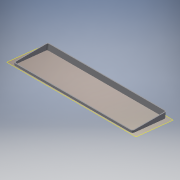
# Autodesk Inventor part: FullEnclosurePrototype2
Saved by Autodesk Inventor 2016 (Build 200138000, 138)
## iProperties
Created: 2021-04-06
Part Number: FullEnclosurePrototype2
Material: Generic
Document SubType Name: Modeling
Designer: Tom
Density: 1 g/cm^3
Appearance: Default
Author: Tom
Autodesk Inventor part; units mm, degrees
(part 1 of 3)
ref_plane "YZ Plane" through (0, 0, 0) normal (1, 0, 0) x (0, 1, 0)
ref_plane "XZ Plane" through (0, 0, 0) normal (0, 1, 0) x (-1, 0, 0)
ref_plane "XY Plane" through (0, 0, 0) normal (0, 0, 1) x (1, 0, 0)
ref_plane "Work Plane1" through (-46.4829, -22.3295, 9.2415) normal (0, 0.1062088, 0.9943439) x (-1, 0, 0)
sketch "Sketch1" plane through (-46.4829, -22.3295, 9.2415) normal (0, 0.1062088, 0.9943439) x (-1, 0, 0)
  line L0 (-256.8052, 108.1981) -> (-256.8112, -5.1571) projected
  ellipse E0 centre (-252.0612, -5.1574) end of major axis (-256.8112, -5.1571) minor radius 4.7231 (-256.8112, -5.1571) -> (-252.0615, -9.8805) ccw projected
  line L1 (-252.0615, -9.8805) -> (180.1885, -9.9036) projected
  ellipse E1 centre (180.1888, -5.1804) end of major axis (175.4388, -5.1802) minor radius 4.7231 (180.1885, -9.9036) -> (184.9388, -5.1807) ccw projected
  line L2 (184.9388, -5.1807) -> (184.9448, 108.1745) projected
  ellipse E2 centre (180.1948, 108.1748) end of major axis (175.4448, 108.175) minor radius 4.7231 (184.9448, 108.1745) -> (180.1951, 112.8979) ccw projected
  line L3 (180.1951, 112.8979) -> (-252.0549, 112.921) projected
  ellipse E3 centre (-252.0552, 108.1978) end of major axis (-256.8052, 108.1981) minor radius 4.7231 (-252.0549, 112.921) -> (-256.8052, 108.1981) ccw projected
  ellipse E4 centre (79.4979, 35.9093) end of major axis (79.2479, 35.9094) minor radius 0.2486 projected
  ellipse E5 centre (81.4737, -6.2143) end of major axis (81.0737, -6.2142) minor radius 0.3977 projected
  ellipse E6 centre (78.9337, -6.2141) end of major axis (78.5337, -6.2141) minor radius 0.3977 projected
  ellipse E7 centre (78.9345, 8.9397) end of major axis (78.5345, 8.9397) minor radius 0.3977 projected
  ellipse E8 centre (78.0659, 35.3197) end of major axis (77.8159, 35.3197) minor radius 0.2486 projected
  ellipse E9 centre (76.6341, 35.9095) end of major axis (76.3841, 35.9095) minor radius 0.2486 projected
  ellipse E10 centre (71.1058, 32.9386) end of major axis (70.3558, 32.9386) minor radius 0.7458 projected
  ellipse E11 centre (68.5655, 27.8874) end of major axis (66.5655, 27.8876) minor radius 1.9887 projected
  ellipse E12 centre (73.6455, 27.8872) end of major axis (72.7955, 27.8872) minor radius 0.8452 projected
  ellipse E13 centre (76.3937, -6.214) end of major axis (75.9937, -6.214) minor radius 0.3977 projected
  ellipse E14 centre (73.8537, -6.2139) end of major axis (73.4537, -6.2138) minor radius 0.3977 projected
  ellipse E15 centre (76.3945, 8.9398) end of major axis (75.9945, 8.9398) minor radius 0.3977 projected
  ellipse E16 centre (71.3137, -6.2137) end of major axis (70.9137, -6.2137) minor radius 0.3977 projected
  ellipse E17 centre (68.7745, 8.9402) end of major axis (68.3745, 8.9402) minor radius 0.3977 projected
  ellipse E18 centre (68.7737, -6.2136) end of major axis (68.3737, -6.2136) minor radius 0.3977 projected
  ellipse E19 centre (43.3737, -6.2122) end of major axis (42.9737, -6.2122) minor radius 0.3977 projected
  ellipse E20 centre (44.9851, 1.469) end of major axis (44.6101, 1.469) minor radius 0.3729 projected
  ellipse E21 centre (44.9852, 2.7318) end of major axis (44.6102, 2.7318) minor radius 0.3729 projected
  ellipse E22 centre (43.3745, 8.9416) end of major axis (42.9745, 8.9416) minor radius 0.3977 projected
  ellipse E23 centre (44.4855, 27.8887) end of major axis (43.6355, 27.8888) minor radius 0.8452 projected
  ellipse E24 centre (50.9937, -6.2126) end of major axis (50.5937, -6.2126) minor radius 0.3977 projected
  ellipse E25 centre (48.4537, -6.2125) end of major axis (48.0537, -6.2125) minor radius 0.3977 projected
  ellipse E26 centre (45.9137, -6.2124) end of major axis (45.5137, -6.2123) minor radius 0.3977 projected
  ellipse E27 centre (56.0737, -6.2129) end of major axis (55.6737, -6.2129) minor radius 0.3977 projected
  ellipse E28 centre (54.891, -1.1616) end of major axis (54.391, -1.1616) minor radius 0.4972 projected
  ellipse E29 centre (53.5337, -6.2128) end of major axis (53.1337, -6.2128) minor radius 0.3977 projected
  ellipse E30 centre (52.3511, 1.3642) end of major axis (51.8511, 1.3642) minor radius 0.4972 projected
  ellipse E31 centre (54.8911, 1.3641) end of major axis (54.3911, 1.3641) minor radius 0.4972 projected
  ellipse E32 centre (58.6137, -6.213) end of major axis (58.2137, -6.213) minor radius 0.3977 projected
  ellipse E33 centre (58.6145, 8.9408) end of major axis (58.2145, 8.9408) minor radius 0.3977 projected
  ellipse E34 centre (53.5345, 8.941) end of major axis (53.1345, 8.941) minor radius 0.3977 projected
  ellipse E35 centre (45.9145, 8.9414) end of major axis (45.5145, 8.9415) minor radius 0.3977 projected
  ellipse E36 centre (48.4545, 8.9413) end of major axis (48.0545, 8.9413) minor radius 0.3977 projected
  ellipse E37 centre (50.9945, 8.9412) end of major axis (50.5945, 8.9412) minor radius 0.3977 projected
  ellipse E38 centre (54.8913, 3.8897) end of major axis (54.3913, 3.8897) minor radius 0.4972 projected
  ellipse E39 centre (54.6455, 27.8882) end of major axis (53.7955, 27.8882) minor radius 0.8452 projected
  ellipse E40 centre (49.5655, 27.8885) end of major axis (47.5655, 27.8886) minor radius 1.9887 projected
  ellipse E41 centre (66.2337, -6.2135) end of major axis (65.8337, -6.2134) minor radius 0.3977 projected
  ellipse E42 centre (63.6937, -6.2133) end of major axis (63.2937, -6.2133) minor radius 0.3977 projected
  ellipse E43 centre (63.6945, 8.9405) end of major axis (63.2945, 8.9405) minor radius 0.3977 projected
  ellipse E44 centre (63.4855, 27.8877) end of major axis (62.6355, 27.8878) minor radius 0.8452 projected
  ellipse E45 centre (61.1537, -6.2132) end of major axis (60.7537, -6.2132) minor radius 0.3977 projected
  ellipse E46 centre (52.1058, 32.9396) end of major axis (51.3558, 32.9396) minor radius 0.7458 projected
  ellipse E47 centre (39.1207, -3.7491) end of major axis (38.8707, -3.7491) minor radius 0.2486 projected
  ellipse E48 centre (39.1206, -6.5967) end of major axis (38.8706, -6.5967) minor radius 0.2486 projected
  ellipse E49 centre (39.7138, -5.1729) end of major axis (39.4638, -5.1729) minor radius 0.2486 projected
  ellipse E50 centre (68.5666, 46.78) end of major axis (66.5666, 46.7801) minor radius 1.9887 projected
  ellipse E51 centre (73.6466, 46.7797) end of major axis (72.7966, 46.7798) minor radius 0.8452 projected
  ellipse E52 centre (80.091, 37.3331) end of major axis (79.841, 37.3331) minor radius 0.2486 projected
  ellipse E53 centre (79.498, 38.7569) end of major axis (79.248, 38.7569) minor radius 0.2486 projected
  ellipse E54 centre (76.6342, 38.7571) end of major axis (76.3842, 38.7571) minor radius 0.2486 projected
  ellipse E55 centre (78.066, 37.3332) end of major axis (76.716, 37.3333) minor radius 1.3424 projected
  ellipse E56 centre (78.0662, 39.3468) end of major axis (77.8162, 39.3468) minor radius 0.2486 projected
  ellipse E57 centre (49.5666, 46.781) end of major axis (47.5666, 46.7811) minor radius 1.9887 projected
  ellipse E58 centre (54.6466, 46.7807) end of major axis (53.7966, 46.7808) minor radius 0.8452 projected
  ellipse E59 centre (63.4866, 46.7803) end of major axis (62.6366, 46.7803) minor radius 0.8452 projected
  ellipse E60 centre (45.7567, 49.3068) end of major axis (45.0067, 49.3069) minor radius 0.7458 projected
  ellipse E61 centre (37.6889, -3.1593) end of major axis (37.4389, -3.1593) minor radius 0.2486 projected
  ellipse E62 centre (36.2568, -6.5966) end of major axis (36.0068, -6.5965) minor radius 0.2486 projected
  ellipse E63 centre (35.6638, -5.1727) end of major axis (35.4138, -5.1727) minor radius 0.2486 projected
  ellipse E64 centre (71.1068, 51.8311) end of major axis (70.3568, 51.8312) minor radius 0.7458 projected
  ellipse E65 centre (52.1068, 51.8321) end of major axis (51.3568, 51.8322) minor radius 0.7458 projected
  ellipse E66 centre (14.8827, 68.201) end of major axis (14.1327, 68.2011) minor radius 0.7458 projected
  ellipse E67 centre (13.6126, 65.6754) end of major axis (12.7626, 65.6755) minor radius 0.8452 projected
  ellipse E68 centre (20.7355, 27.89) end of major axis (19.8855, 27.89) minor radius 0.8452 projected
  ellipse E69 centre (22.0057, 30.4156) end of major axis (21.2557, 30.4156) minor radius 0.7458 projected
  ellipse E70 centre (21.0666, 46.7825) end of major axis (19.0666, 46.7826) minor radius 1.9887 projected
  ellipse E71 centre (29.1358, 68.974) end of major axis (28.8858, 68.974) minor radius 0.2486 projected
  ellipse E72 centre (23.7726, 65.6749) end of major axis (22.9226, 65.675) minor radius 0.8452 projected
  ellipse E73 centre (28.3543, 4.6021) end of major axis (27.6043, 4.6021) minor radius 0.7458 projected
  ellipse E74 centre (25.814, -0.4491) end of major axis (23.814, -0.449) minor radius 1.9887 projected
  ellipse E75 centre (20.734, -0.4488) end of major axis (19.884, -0.4488) minor radius 0.8452 projected
  ellipse E76 centre (30.5677, 68.3841) end of major axis (30.3177, 68.3841) minor radius 0.2486 projected
  ellipse E77 centre (5.2939, -3.3316) end of major axis (4.8939, -3.3316) minor radius 0.3977 projected
  ellipse E78 centre (7.8939, -3.3317) end of major axis (7.4939, -3.3317) minor radius 0.3977 projected
  ellipse E79 centre (5.5937, -6.9609) end of major axis (5.0937, -6.9609) minor radius 0.4972 (5.5937, -6.4638) -> (5.5937, -7.4581) ccw projected
  line L4 (7.5937, -6.4639) -> (5.5937, -6.4638) projected
  ellipse E80 centre (7.5937, -6.961) end of major axis (7.0937, -6.961) minor radius 0.4972 (7.5937, -7.4582) -> (7.5937, -6.4639) ccw projected
  line L5 (5.5937, -7.4581) -> (7.5937, -7.4582) projected
  ellipse E81 centre (9.994, -0.5477) end of major axis (9.594, -0.5476) minor radius 0.3977 projected
  ellipse E82 centre (9.1913, 41.712) end of major axis (8.9413, 41.712) minor radius 0.2486 projected
  ellipse E83 centre (9.1912, 39.6985) end of major axis (7.8412, 39.6985) minor radius 1.3424 projected
  ellipse E84 centre (7.7594, 41.1223) end of major axis (7.5094, 41.1223) minor radius 0.2486 projected
  ellipse E85 centre (10.623, 38.2746) end of major axis (10.373, 38.2746) minor radius 0.2486 projected
  ellipse E86 centre (9.1911, 37.6849) end of major axis (8.9411, 37.6849) minor radius 0.2486 projected
  ellipse E87 centre (9.3558, 32.9419) end of major axis (8.6058, 32.9419) minor radius 0.7458 projected
  line L6 (13.9437, -6.9117) -> (13.9438, -5.4202) projected
  ellipse E88 centre (13.4437, -6.9116) end of major axis (12.9437, -6.9116) minor radius 0.4972 (12.9437, -6.9116) -> (13.9437, -6.9117) ccw projected
  line L7 (12.9438, -5.4201) -> (12.9437, -6.9116) projected
  ellipse E89 centre (13.4438, -5.4201) end of major axis (12.9438, -5.4201) minor radius 0.4972 (13.9438, -5.4202) -> (12.9438, -5.4201) ccw projected
  ellipse E90 centre (11.2162, 39.6983) end of major axis (10.9662, 39.6984) minor radius 0.2486 projected
  ellipse E91 centre (37.6887, -7.1864) end of major axis (37.4387, -7.1864) minor radius 0.2486 projected
  ellipse E92 centre (37.6888, -5.1728) end of major axis (36.3388, -5.1728) minor radius 1.3424 projected
  ellipse E93 centre (30.894, -0.4493) end of major axis (30.044, -0.4493) minor radius 0.8452 projected
  ellipse E94 centre (25.8155, 27.8897) end of major axis (23.8155, 27.8898) minor radius 1.9887 projected
  ellipse E95 centre (30.8955, 27.8895) end of major axis (30.0455, 27.8895) minor radius 0.8452 projected
  ellipse E96 centre (22.0042, 2.0768) end of major axis (21.2542, 2.0768) minor radius 0.7458 projected
  ellipse E97 centre (-36.2645, 27.893) end of major axis (-37.1145, 27.8931) minor radius 0.8452 projected
  ellipse E98 centre (-34.9943, 30.4186) end of major axis (-35.7443, 30.4186) minor radius 0.7458 projected
  ellipse E99 centre (-28.6442, 32.9439) end of major axis (-29.3942, 32.9439) minor radius 0.7458 projected
  ellipse E100 centre (-31.1845, 27.8928) end of major axis (-33.1845, 27.8929) minor radius 1.9887 projected
  ellipse E101 centre (-26.7634, 46.7851) end of major axis (-27.6134, 46.7851) minor radius 0.8452 projected
  ellipse E102 centre (-15.9943, 30.4176) end of major axis (-16.7443, 30.4176) minor radius 0.7458 projected
  ellipse E103 centre (-17.2645, 27.892) end of major axis (-18.1145, 27.8921) minor radius 0.8452 projected
  ellipse E104 centre (-21.6834, 46.7848) end of major axis (-23.6834, 46.7849) minor radius 1.9887 projected
  ellipse E105 centre (-25.4933, 49.3106) end of major axis (-26.2433, 49.3107) minor radius 0.7458 projected
  ellipse E106 centre (-12.1845, 27.8918) end of major axis (-14.1845, 27.8919) minor radius 1.9887 projected
  ellipse E107 centre (-9.6442, 32.9429) end of major axis (-10.3942, 32.9429) minor radius 0.7458 projected
  ellipse E108 centre (-12.186, -0.447) end of major axis (-14.186, -0.4469) minor radius 1.9887 projected
  ellipse E109 centre (-28.6457, 4.6051) end of major axis (-29.3957, 4.6051) minor radius 0.7458 projected
  ellipse E110 centre (-31.186, -0.446) end of major axis (-33.186, -0.4459) minor radius 1.9887 projected
  ellipse E111 centre (-19.1432, 51.8359) end of major axis (-19.8932, 51.836) minor radius 0.7458 projected
  ellipse E112 centre (-7.106, -0.4473) end of major axis (-7.956, -0.4473) minor radius 0.8452 projected
  ellipse E113 centre (-6.4933, 49.3096) end of major axis (-7.2433, 49.3097) minor radius 0.7458 projected
  ellipse E114 centre (-7.7634, 46.7841) end of major axis (-8.6134, 46.7841) minor radius 0.8452 projected
  ellipse E115 centre (-0.2562, -5.4194) end of major axis (-0.7562, -5.4194) minor radius 0.4972 (0.2438, -5.4194) -> (-0.7562, -5.4194) ccw projected
  line L8 (0.2437, -6.9109) -> (0.2438, -5.4194) projected
  ellipse E116 centre (-0.2563, -6.9109) end of major axis (-0.7563, -6.9109) minor radius 0.4972 (-0.7563, -6.9109) -> (0.2437, -6.9109) ccw projected
  line L9 (-0.7562, -5.4194) -> (-0.7563, -6.9109) projected
  ellipse E117 centre (-2.6834, 46.7838) end of major axis (-4.6834, 46.7839) minor radius 1.9887 projected
  ellipse E118 centre (-11.2423, 68.2024) end of major axis (-11.9923, 68.2024) minor radius 0.7458 projected
  ellipse E119 centre (-12.5124, 65.6768) end of major axis (-13.3624, 65.6769) minor radius 0.8452 projected
  ellipse E120 centre (-7.4324, 65.6766) end of major axis (-9.4324, 65.6767) minor radius 1.9887 projected
  ellipse E121 centre (-30.2423, 68.2034) end of major axis (-30.9923, 68.2035) minor radius 0.7458 projected
  ellipse E122 centre (-31.5124, 65.6779) end of major axis (-32.3624, 65.6779) minor radius 0.8452 projected
  ellipse E123 centre (1.7355, 27.891) end of major axis (0.8855, 27.8911) minor radius 0.8452 projected
  ellipse E124 centre (3.0057, 30.4166) end of major axis (2.2557, 30.4166) minor radius 0.7458 projected
  ellipse E125 centre (2.3966, 46.7835) end of major axis (1.5466, 46.7836) minor radius 0.8452 projected
  ellipse E126 centre (3.1939, -3.3315) end of major axis (2.7939, -3.3314) minor radius 0.3977 projected
  ellipse E127 centre (3.194, -0.5473) end of major axis (2.794, -0.5473) minor radius 0.3977 projected
  ellipse E128 centre (-4.8922, 70.7277) end of major axis (-5.6422, 70.7277) minor radius 0.7458 projected
  ellipse E129 centre (-23.8922, 70.7287) end of major axis (-24.6422, 70.7288) minor radius 0.7458 projected
  ellipse E130 centre (-24.9999, 77.1501) end of major axis (-25.2499, 77.1502) minor radius 0.2486 projected
  ellipse E131 centre (-27.8637, 77.1503) end of major axis (-28.1137, 77.1503) minor radius 0.2486 projected
  ellipse E132 centre (-24.4069, 75.7263) end of major axis (-24.6569, 75.7263) minor radius 0.2486 projected
  ellipse E133 centre (-25.0001, 74.3026) end of major axis (-25.2501, 74.3026) minor radius 0.2486 projected
  ellipse E134 centre (-28.4569, 75.7265) end of major axis (-28.7069, 75.7265) minor radius 0.2486 projected
  ellipse E135 centre (-26.432, 73.7129) end of major axis (-26.682, 73.7129) minor radius 0.2486 projected
  ellipse E136 centre (29.136, 71.8215) end of major axis (28.886, 71.8216) minor radius 0.2486 projected
  ellipse E137 centre (30.5679, 72.4112) end of major axis (30.3179, 72.4112) minor radius 0.2486 projected
  ellipse E138 centre (8.8636, 84.5682) end of major axis (8.0136, 84.5683) minor radius 0.8452 projected
  ellipse E139 centre (-11.8514, 84.5693) end of major axis (-12.7014, 84.5694) minor radius 0.8452 projected
  ellipse E140 centre (19.0236, 84.5677) end of major axis (18.1736, 84.5677) minor radius 0.8452 projected
  ellipse E141 centre (68.5686, 84.565) end of major axis (66.5686, 84.5652) minor radius 1.9887 projected
  ellipse E142 centre (-30.8514, 84.5704) end of major axis (-31.7014, 84.5704) minor radius 0.8452 projected
  ellipse E143 centre (-22.0114, 84.5699) end of major axis (-22.8614, 84.5699) minor radius 0.8452 projected
  ellipse E144 centre (-26.4318, 77.74) end of major axis (-26.6818, 77.74) minor radius 0.2486 projected
  ellipse E145 centre (64.7587, 87.0909) end of major axis (64.0087, 87.0909) minor radius 0.7458 projected
  ellipse E146 centre (-144.8514, 84.5764) end of major axis (-145.7014, 84.5765) minor radius 0.8452 projected
  ellipse E147 centre (-145.5124, 65.6839) end of major axis (-146.3624, 65.684) minor radius 0.8452 projected
  ellipse E148 centre (-145.1838, 40.1144) end of major axis (-145.4338, 40.1144) minor radius 0.2486 projected
  ellipse E149 centre (-140.7634, 46.7912) end of major axis (-141.6134, 46.7912) minor radius 0.8452 projected
  ellipse E150 centre (-134.7413, 87.1015) end of major axis (-135.4913, 87.1016) minor radius 0.7458 projected
  ellipse E151 centre (-136.0114, 84.576) end of major axis (-136.8614, 84.576) minor radius 0.8452 projected
  ellipse E152 centre (-135.6834, 46.7909) end of major axis (-137.6834, 46.791) minor radius 1.9887 projected
  ellipse E153 centre (-116.6834, 46.7899) end of major axis (-118.6834, 46.79) minor radius 1.9887 projected
  ellipse E154 centre (-114.1432, 51.841) end of major axis (-114.8932, 51.841) minor radius 0.7458 projected
  ellipse E155 centre (-116.3524, 65.6824) end of major axis (-117.2024, 65.6824) minor radius 0.8452 projected
  ellipse E156 centre (-120.4933, 49.3157) end of major axis (-121.2433, 49.3157) minor radius 0.7458 projected
  ellipse E157 centre (-121.4324, 65.6827) end of major axis (-123.4324, 65.6828) minor radius 1.9887 projected
  ellipse E158 centre (-125.8514, 84.5754) end of major axis (-126.7014, 84.5755) minor radius 0.8452 projected
  ellipse E159 centre (-111.9314, 84.5747) end of major axis (-113.9314, 84.5748) minor radius 1.9887 projected
  ellipse E160 centre (-111.9319, 76.4817) end of major axis (-112.1819, 76.4817) minor radius 0.2486 projected
  ellipse E161 centre (-113.3639, 73.0445) end of major axis (-113.6139, 73.0445) minor radius 0.2486 projected
  ellipse E162 centre (-125.2423, 68.2085) end of major axis (-125.9923, 68.2085) minor radius 0.7458 projected
  ellipse E163 centre (-130.6034, 46.7906) end of major axis (-131.4534, 46.7907) minor radius 0.8452 projected
  ellipse E164 centre (-92.9314, 84.5737) end of major axis (-94.9314, 84.5738) minor radius 1.9887 projected
  ellipse E165 centre (-98.0114, 84.5739) end of major axis (-98.8614, 84.574) minor radius 0.8452 projected
  ellipse E166 centre (-99.8922, 70.7328) end of major axis (-100.6422, 70.7328) minor radius 0.7458 projected
  ellipse E167 centre (-101.4933, 49.3147) end of major axis (-102.2433, 49.3147) minor radius 0.7458 projected
  ellipse E168 centre (-95.1432, 51.84) end of major axis (-95.8932, 51.84) minor radius 0.7458 projected
  ellipse E169 centre (-97.3524, 65.6814) end of major axis (-98.2024, 65.6814) minor radius 0.8452 projected
  ellipse E170 centre (-106.2423, 68.2075) end of major axis (-106.9923, 68.2075) minor radius 0.7458 projected
  ellipse E171 centre (-106.8514, 84.5744) end of major axis (-107.7014, 84.5745) minor radius 0.8452 projected
  ellipse E172 centre (-107.5124, 65.6819) end of major axis (-108.3624, 65.682) minor radius 0.8452 projected
  ellipse E173 centre (-145.184, 36.0873) end of major axis (-145.434, 36.0873) minor radius 0.2486 projected
  ellipse E174 centre (-143.1589, 38.1007) end of major axis (-143.4089, 38.1007) minor radius 0.2486 projected
  ellipse E175 centre (-142.6442, 32.95) end of major axis (-143.3942, 32.95) minor radius 0.7458 projected
  ellipse E176 centre (-87.8514, 84.5734) end of major axis (-88.7014, 84.5734) minor radius 0.8452 projected
  ellipse E177 centre (-82.0043, -3.7427) end of major axis (-82.2543, -3.7426) minor radius 0.2486 projected
  ellipse E178 centre (-84.868, -3.7425) end of major axis (-85.118, -3.7425) minor radius 0.2486 projected
  ellipse E179 centre (-101.4958, 2.0834) end of major axis (-102.2458, 2.0834) minor radius 0.7458 projected
  ellipse E180 centre (-83.7634, 46.7881) end of major axis (-84.6134, 46.7882) minor radius 0.8452 projected
  ellipse E181 centre (-97.6834, 46.7889) end of major axis (-99.6834, 46.789) minor radius 1.9887 projected
  ellipse E182 centre (-102.7634, 46.7891) end of major axis (-103.6134, 46.7892) minor radius 0.8452 projected
  ellipse E183 centre (-102.1045, 27.8966) end of major axis (-102.9545, 27.8966) minor radius 0.8452 projected
  ellipse E184 centre (-91.9943, 30.4217) end of major axis (-92.7443, 30.4217) minor radius 0.7458 projected
  ellipse E185 centre (-93.2645, 27.8961) end of major axis (-94.1145, 27.8961) minor radius 0.8452 projected
  ellipse E186 centre (-88.1845, 27.8958) end of major axis (-90.1845, 27.8959) minor radius 1.9887 projected
  ellipse E187 centre (-83.1045, 27.8955) end of major axis (-83.9545, 27.8956) minor radius 0.8452 projected
  ellipse E188 centre (-121.1045, 27.8976) end of major axis (-121.9545, 27.8976) minor radius 0.8452 projected
  ellipse E189 centre (-121.7634, 46.7901) end of major axis (-122.6134, 46.7902) minor radius 0.8452 projected
  ellipse E190 centre (-116.686, -0.4415) end of major axis (-118.686, -0.4414) minor radius 1.9887 projected
  ellipse E191 centre (-120.4958, 2.0844) end of major axis (-121.2458, 2.0844) minor radius 0.7458 projected
  ellipse E192 centre (-121.766, -0.4412) end of major axis (-122.616, -0.4411) minor radius 0.8452 projected
  ellipse E193 centre (-114.1457, 4.6097) end of major axis (-114.8957, 4.6097) minor radius 0.7458 projected
  ellipse E194 centre (-111.6034, 46.7896) end of major axis (-112.4534, 46.7896) minor radius 0.8452 projected
  ellipse E195 centre (-110.9943, 30.4227) end of major axis (-111.7443, 30.4227) minor radius 0.7458 projected
  ellipse E196 centre (-111.606, -0.4417) end of major axis (-112.456, -0.4417) minor radius 0.8452 projected
  ellipse E197 centre (-104.6442, 32.948) end of major axis (-105.3942, 32.948) minor radius 0.7458 projected
  ellipse E198 centre (-133.1457, 4.6107) end of major axis (-133.8957, 4.6107) minor radius 0.7458 projected
  ellipse E199 centre (-135.686, -0.4404) end of major axis (-137.686, -0.4403) minor radius 1.9887 projected
  ellipse E200 centre (-130.606, -0.4407) end of major axis (-131.456, -0.4407) minor radius 0.8452 projected
  ellipse E201 centre (-126.1845, 27.8978) end of major axis (-128.1845, 27.898) minor radius 1.9887 projected
  ellipse E202 centre (-123.6442, 32.949) end of major axis (-124.3942, 32.949) minor radius 0.7458 projected
  ellipse E203 centre (-140.766, -0.4402) end of major axis (-141.616, -0.4401) minor radius 0.8452 projected
  ellipse E204 centre (-74.266, -0.4437) end of major axis (-75.116, -0.4437) minor radius 0.8452 projected
  ellipse E205 centre (-72.9943, 30.4206) end of major axis (-73.7443, 30.4207) minor radius 0.7458 projected
  ellipse E206 centre (-74.2645, 27.8951) end of major axis (-75.1145, 27.8951) minor radius 0.8452 projected
  ellipse E207 centre (-79.0114, 84.5729) end of major axis (-79.8614, 84.573) minor radius 0.8452 projected
  ellipse E208 centre (-73.6034, 46.7876) end of major axis (-74.4534, 46.7876) minor radius 0.8452 projected
  ellipse E209 centre (-78.6834, 46.7878) end of major axis (-80.6834, 46.7879) minor radius 1.9887 projected
  ellipse E210 centre (-80.8922, 70.7318) end of major axis (-81.6422, 70.7318) minor radius 0.7458 projected
  ellipse E211 centre (-83.4324, 65.6806) end of major axis (-85.4324, 65.6807) minor radius 1.9887 projected
  ellipse E212 centre (-85.6442, 32.9469) end of major axis (-86.3942, 32.947) minor radius 0.7458 projected
  ellipse E213 centre (-77.7413, 87.0985) end of major axis (-78.4913, 87.0985) minor radius 0.7458 projected
  ellipse E214 centre (-55.2645, 27.8941) end of major axis (-56.1145, 27.8941) minor radius 0.8452 projected
  ellipse E215 centre (-53.9943, 30.4196) end of major axis (-54.7443, 30.4197) minor radius 0.7458 projected
  ellipse E216 centre (-69.1845, 27.8948) end of major axis (-71.1845, 27.8949) minor radius 1.9887 projected
  ellipse E217 centre (-64.1045, 27.8945) end of major axis (-64.9545, 27.8946) minor radius 0.8452 projected
  ellipse E218 centre (-67.1589, 38.0967) end of major axis (-67.4089, 38.0967) minor radius 0.2486 projected
  ellipse E219 centre (-70.6159, 36.6731) end of major axis (-70.8659, 36.6731) minor radius 0.2486 projected
  ellipse E220 centre (-71.2089, 38.0969) end of major axis (-71.4589, 38.0969) minor radius 0.2486 projected
  ellipse E221 centre (-66.6442, 32.9459) end of major axis (-67.3942, 32.946) minor radius 0.7458 projected
  ellipse E222 centre (-70.6157, 39.5206) end of major axis (-70.8657, 39.5207) minor radius 0.2486 projected
  ellipse E223 centre (-67.7519, 39.5205) end of major axis (-68.0019, 39.5205) minor radius 0.2486 projected
  ellipse E224 centre (-53.9958, 2.0808) end of major axis (-54.7458, 2.0809) minor radius 0.7458 projected
  ellipse E225 centre (-64.106, -0.4443) end of major axis (-64.956, -0.4442) minor radius 0.8452 projected
  ellipse E226 centre (-55.266, -0.4447) end of major axis (-56.116, -0.4447) minor radius 0.8452 projected
  ellipse E227 centre (-54.9314, 84.5716) end of major axis (-56.9314, 84.5717) minor radius 1.9887 projected
  ellipse E228 centre (-60.0114, 84.5719) end of major axis (-60.8614, 84.572) minor radius 0.8452 projected
  ellipse E229 centre (-59.6834, 46.7868) end of major axis (-61.6834, 46.7869) minor radius 1.9887 projected
  ellipse E230 centre (-59.3524, 65.6793) end of major axis (-60.2024, 65.6794) minor radius 0.8452 projected
  ellipse E231 centre (-64.4324, 65.6796) end of major axis (-66.4324, 65.6797) minor radius 1.9887 projected
  ellipse E232 centre (-63.4933, 49.3127) end of major axis (-64.2433, 49.3127) minor radius 0.7458 projected
  ellipse E233 centre (-84.8682, -6.5901) end of major axis (-85.1182, -6.5901) minor radius 0.2486 projected
  ellipse E234 centre (-85.4612, -5.1663) end of major axis (-85.7112, -5.1662) minor radius 0.2486 projected
  ellipse E235 centre (-82.0044, -6.5902) end of major axis (-82.2544, -6.5902) minor radius 0.2486 projected
  ellipse E236 centre (-83.4362, -5.1664) end of major axis (-84.7862, -5.1663) minor radius 1.3424 projected
  ellipse E237 centre (-81.4112, -5.1665) end of major axis (-81.6612, -5.1665) minor radius 0.2486 projected
  ellipse E238 centre (-38.1432, 51.8369) end of major axis (-38.8932, 51.837) minor radius 0.7458 projected
  ellipse E239 centre (-44.4933, 49.3116) end of major axis (-45.2433, 49.3117) minor radius 0.7458 projected
  ellipse E240 centre (-47.6442, 32.9449) end of major axis (-48.3942, 32.945) minor radius 0.7458 projected
  ellipse E241 centre (-45.1045, 27.8935) end of major axis (-45.9545, 27.8936) minor radius 0.8452 projected
  ellipse E242 centre (-50.186, -0.445) end of major axis (-52.186, -0.4449) minor radius 1.9887 projected
  ellipse E243 centre (-47.6457, 4.6061) end of major axis (-48.3957, 4.6062) minor radius 0.7458 projected
  ellipse E244 centre (-45.106, -0.4453) end of major axis (-45.956, -0.4452) minor radius 0.8452 projected
  ellipse E245 centre (-49.8514, 84.5714) end of major axis (-50.7014, 84.5714) minor radius 0.8452 projected
  ellipse E246 centre (-41.0114, 84.5709) end of major axis (-41.8614, 84.5709) minor radius 0.8452 projected
  ellipse E247 centre (-83.4363, -7.1799) end of major axis (-83.6863, -7.1799) minor radius 0.2486 projected
  ellipse E248 centre (144.2376, 65.6685) end of major axis (143.3876, 65.6685) minor radius 0.8452 projected
  ellipse E249 centre (135.3976, 65.6689) end of major axis (134.5476, 65.669) minor radius 0.8452 projected
  ellipse E250 centre (130.3166, 46.7767) end of major axis (128.3166, 46.7768) minor radius 1.9887 projected
  ellipse E251 centre (144.2366, 46.7759) end of major axis (143.3866, 46.776) minor radius 0.8452 projected
  ellipse E252 centre (145.5067, 49.3015) end of major axis (144.7567, 49.3015) minor radius 0.7458 projected
  ellipse E253 centre (130.3155, 27.8842) end of major axis (128.3155, 27.8843) minor radius 1.9887 projected
  ellipse E254 centre (132.8558, 32.9353) end of major axis (132.1058, 32.9353) minor radius 0.7458 projected
  ellipse E255 centre (138.3842, 38.7538) end of major axis (138.1342, 38.7538) minor radius 0.2486 projected
  ellipse E256 centre (144.2355, 27.8834) end of major axis (143.3855, 27.8835) minor radius 0.8452 projected
  ellipse E257 centre (145.5057, 30.409) end of major axis (144.7557, 30.409) minor radius 0.7458 projected
  ellipse E258 centre (141.2479, 35.906) end of major axis (140.9979, 35.9061) minor radius 0.2486 projected
  ellipse E259 centre (139.8162, 39.3435) end of major axis (139.5662, 39.3435) minor radius 0.2486 projected
  ellipse E260 centre (118.3164, 44.3909) end of major axis (116.7914, 44.391) minor radius 1.5164 projected
  ellipse E261 centre (116.3955, 27.8849) end of major axis (115.5455, 27.8849) minor radius 0.8452 projected
  ellipse E262 centre (116.3971, 56.2237) end of major axis (115.5471, 56.2237) minor radius 0.8452 projected
  ellipse E263 centre (83.7557, 30.4123) end of major axis (83.0057, 30.4123) minor radius 0.7458 projected
  ellipse E264 centre (82.4855, 27.8867) end of major axis (81.6355, 27.8867) minor radius 0.8452 projected
  ellipse E265 centre (87.5655, 27.8864) end of major axis (85.5655, 27.8865) minor radius 1.9887 projected
  ellipse E266 centre (90.1058, 32.9376) end of major axis (89.3558, 32.9376) minor radius 0.7458 projected
  ellipse E267 centre (92.6455, 27.8862) end of major axis (91.7955, 27.8862) minor radius 0.8452 projected
  ellipse E268 centre (111.3155, 27.8852) end of major axis (109.3155, 27.8853) minor radius 1.9887 projected
  ellipse E269 centre (113.8558, 32.9363) end of major axis (113.1058, 32.9363) minor radius 0.7458 projected
  ellipse E270 centre (107.5057, 30.411) end of major axis (106.7557, 30.411) minor radius 0.7458 projected
  ellipse E271 centre (103.0777, 68.0571) end of major axis (101.0777, 68.0572) minor radius 1.9887 projected
  ellipse E272 centre (83.7567, 49.3048) end of major axis (83.0067, 49.3048) minor radius 0.7458 projected
  ellipse E273 centre (82.4866, 46.7792) end of major axis (81.6366, 46.7793) minor radius 0.8452 projected
  ellipse E274 centre (87.5666, 46.779) end of major axis (85.5666, 46.7791) minor radius 1.9887 projected
  ellipse E275 centre (90.1068, 51.8301) end of major axis (89.3568, 51.8301) minor radius 0.7458 projected
  ellipse E276 centre (92.6466, 46.7787) end of major axis (91.7966, 46.7787) minor radius 0.8452 projected
  ellipse E277 centre (107.5072, 58.7498) end of major axis (106.7572, 58.7498) minor radius 0.7458 projected
  ellipse E278 centre (106.2371, 56.2242) end of major axis (105.3871, 56.2243) minor radius 0.8452 projected
  ellipse E279 centre (111.3171, 56.224) end of major axis (109.3171, 56.2241) minor radius 1.9887 projected
  ellipse E280 centre (132.8578, 70.7203) end of major axis (132.1078, 70.7204) minor radius 0.7458 projected
  ellipse E281 centre (130.3186, 84.5617) end of major axis (128.3186, 84.5619) minor radius 1.9887 projected
  ellipse E282 centre (137.7931, 75.1151) end of major axis (137.5431, 75.1151) minor radius 0.2486 projected
  ellipse E283 centre (125.2386, 84.562) end of major axis (124.3886, 84.5621) minor radius 0.8452 projected
  ellipse E284 centre (118.3184, 82.176) end of major axis (116.7934, 82.176) minor radius 1.5164 projected
  ellipse E285 centre (141.2499, 73.6911) end of major axis (140.9999, 73.6911) minor radius 0.2486 projected
  ellipse E286 centre (103.0784, 82.1768) end of major axis (101.0784, 82.1769) minor radius 1.9887 projected
  ellipse E287 centre (84.0137, -6.2144) end of major axis (83.6137, -6.2144) minor radius 0.3977 projected
  ellipse E288 centre (86.5537, -6.2145) end of major axis (86.1537, -6.2145) minor radius 0.3977 projected
  ellipse E289 centre (86.5545, 8.9393) end of major axis (86.1545, 8.9393) minor radius 0.3977 projected
  ellipse E290 centre (84.0145, 8.9394) end of major axis (83.6145, 8.9394) minor radius 0.3977 projected
  ellipse E291 centre (89.0937, -6.2147) end of major axis (88.6937, -6.2146) minor radius 0.3977 projected
  ellipse E292 centre (89.0945, 8.9391) end of major axis (88.6945, 8.9392) minor radius 0.3977 projected
  ellipse E293 centre (91.6345, 8.939) end of major axis (91.2345, 8.939) minor radius 0.3977 projected
  ellipse E294 centre (91.6337, -6.2148) end of major axis (91.2337, -6.2148) minor radius 0.3977 projected
  ellipse E295 centre (-154.686, -0.4394) end of major axis (-156.686, -0.4393) minor radius 1.9887 projected
  ellipse E296 centre (-152.1432, 51.843) end of major axis (-152.8932, 51.8431) minor radius 0.7458 projected
  ellipse E297 centre (-154.6834, 46.7919) end of major axis (-156.6834, 46.792) minor radius 1.9887 projected
  ellipse E298 centre (-146.6159, 36.6771) end of major axis (-146.8659, 36.6771) minor radius 0.2486 projected
  ellipse E299 centre (-145.1839, 38.1008) end of major axis (-146.5339, 38.1009) minor radius 1.3424 projected
  ellipse E300 centre (-146.6157, 39.5247) end of major axis (-146.8657, 39.5247) minor radius 0.2486 projected
  ellipse E301 centre (-143.7521, 36.677) end of major axis (-144.0021, 36.677) minor radius 0.2486 projected
  ellipse E302 centre (-143.7519, 39.5245) end of major axis (-144.0019, 39.5246) minor radius 0.2486 projected
  ellipse E303 centre (-147.2089, 38.1009) end of major axis (-147.4589, 38.1009) minor radius 0.2486 projected
  ellipse E304 centre (-150.2645, 27.8991) end of major axis (-151.1145, 27.8992) minor radius 0.8452 projected
  ellipse E305 centre (-145.1845, 27.8989) end of major axis (-147.1845, 27.899) minor radius 1.9887 projected
  ellipse E306 centre (-149.606, -0.4397) end of major axis (-150.456, -0.4397) minor radius 0.8452 projected
  ellipse E307 centre (-154.3524, 65.6844) end of major axis (-155.2024, 65.6845) minor radius 0.8452 projected
  ellipse E308 centre (-155.0114, 84.577) end of major axis (-155.8614, 84.577) minor radius 0.8452 projected
  ellipse E309 centre (173.3955, 27.8819) end of major axis (172.5455, 27.8819) minor radius 0.8452 projected
  ellipse E310 centre (163.2355, 27.8824) end of major axis (162.3855, 27.8824) minor radius 0.8452 projected
  ellipse E311 centre (170.8558, 32.9333) end of major axis (170.1058, 32.9333) minor radius 0.7458 projected
  ellipse E312 centre (164.5057, 30.408) end of major axis (163.7557, 30.408) minor radius 0.7458 projected
  ellipse E313 centre (168.3166, 46.7747) end of major axis (166.3166, 46.7748) minor radius 1.9887 projected
  ellipse E314 centre (164.5077, 68.193) end of major axis (163.7577, 68.1931) minor radius 0.7458 projected
  ellipse E315 centre (163.2376, 65.6675) end of major axis (162.3876, 65.6675) minor radius 0.8452 projected
  ellipse E316 centre (164.5067, 49.3005) end of major axis (163.7567, 49.3005) minor radius 0.7458 projected
  ellipse E317 centre (163.2366, 46.7749) end of major axis (162.3866, 46.775) minor radius 0.8452 projected
  ellipse E318 centre (170.8568, 51.8258) end of major axis (170.1068, 51.8258) minor radius 0.7458 projected
  ellipse E319 centre (170.8578, 70.7183) end of major axis (170.1078, 70.7184) minor radius 0.7458 projected
  ellipse E320 centre (154.3976, 65.6679) end of major axis (153.5476, 65.668) minor radius 0.8452 projected
  ellipse E321 centre (154.3955, 27.8829) end of major axis (153.5455, 27.8829) minor radius 0.8452 projected
  ellipse E322 centre (149.3166, 46.7757) end of major axis (147.3166, 46.7758) minor radius 1.9887 projected
  ellipse E323 centre (151.8568, 51.8268) end of major axis (151.1068, 51.8268) minor radius 0.7458 projected
  ellipse E324 centre (151.8578, 70.7193) end of major axis (151.1078, 70.7194) minor radius 0.7458 projected
  ellipse E325 centre (154.3986, 84.5605) end of major axis (153.5486, 84.5605) minor radius 0.8452 projected
  ellipse E326 centre (173.3986, 84.5595) end of major axis (172.5486, 84.5595) minor radius 0.8452 projected
  ellipse E327 centre (164.5087, 87.0856) end of major axis (163.7587, 87.0856) minor radius 0.7458 projected
  ellipse E328 centre (49.5696, 103.4586) end of major axis (47.5696, 103.4587) minor radius 1.9887 projected
  ellipse E329 centre (28.5246, 103.4597) end of major axis (27.6746, 103.4598) minor radius 0.8452 projected
  ellipse E330 centre (18.3646, 103.4603) end of major axis (17.5146, 103.4603) minor radius 0.8452 projected
  ellipse E331 centre (-50.0309, 95.2705) end of major axis (-52.0309, 95.2706) minor radius 1.9887 projected
  ellipse E332 centre (-24.0554, 103.4625) end of major axis (-26.0554, 103.4626) minor radius 1.9887 projected
  ellipse E333 centre (2.0439, 91.529) end of major axis (0.5189, 91.5291) minor radius 1.5164 projected
  ellipse E334 centre (-52.3912, 89.6228) end of major axis (-53.1412, 89.6228) minor radius 0.7458 projected
  ellipse E335 centre (-33.3912, 89.6218) end of major axis (-34.1412, 89.6218) minor radius 0.7458 projected
  ellipse E336 centre (16.4838, 89.6191) end of major axis (15.7338, 89.6191) minor radius 0.7458 projected
  ellipse E337 centre (113.8593, 99.0602) end of major axis (113.1093, 99.0602) minor radius 0.7458 projected
  ellipse E338 centre (111.3191, 94.009) end of major axis (109.3191, 94.0091) minor radius 1.9887 projected
  ellipse E339 centre (106.2391, 94.0093) end of major axis (105.3891, 94.0093) minor radius 0.8452 projected
  ellipse E340 centre (71.1088, 89.6162) end of major axis (70.3588, 89.6162) minor radius 0.7458 projected
  ellipse E341 centre (103.0797, 105.8422) end of major axis (101.0797, 105.8423) minor radius 1.9887 projected
  ellipse E342 centre (170.8588, 89.6109) end of major axis (170.1088, 89.6109) minor radius 0.7458 projected
  ellipse E343 centre (151.8588, 89.6119) end of major axis (151.1088, 89.6119) minor radius 0.7458 projected
  ellipse E344 centre (126.5097, 105.9801) end of major axis (125.7597, 105.9802) minor radius 0.7458 projected
  ellipse E345 centre (130.3196, 103.4543) end of major axis (128.3196, 103.4544) minor radius 1.9887 projected
  ellipse E346 centre (144.2396, 103.4535) end of major axis (143.3896, 103.4536) minor radius 0.8452 projected
  ellipse E347 centre (135.3996, 103.454) end of major axis (134.5496, 103.4541) minor radius 0.8452 projected
  ellipse E348 centre (-128.3912, 89.6268) end of major axis (-129.1412, 89.6269) minor radius 0.7458 projected
  ellipse E349 centre (-107.1804, 103.467) end of major axis (-109.1804, 103.4671) minor radius 1.9887 projected
  ellipse E350 centre (-109.3912, 89.6258) end of major axis (-110.1412, 89.6259) minor radius 0.7458 projected
  ellipse E351 centre (-61.1121, 106.7638) end of major axis (-61.3621, 106.7639) minor radius 0.2486 projected
  ellipse E352 centre (-147.3912, 89.6278) end of major axis (-148.1412, 89.6279) minor radius 0.7458 projected
  ellipse E353 centre (-218.7841, 34.8632) end of major axis (-220.3091, 34.8633) minor radius 1.5164 projected
  ellipse E354 centre (-199.6442, 32.953) end of major axis (-200.3942, 32.9531) minor radius 0.7458 projected
  ellipse E355 centre (-161.6442, 32.951) end of major axis (-162.3942, 32.951) minor radius 0.7458 projected
  ellipse E356 centre (-180.6442, 32.952) end of major axis (-181.3942, 32.9521) minor radius 0.7458 projected
  ellipse E357 centre (-215.4933, 49.3208) end of major axis (-216.2433, 49.3208) minor radius 0.7458 projected
  ellipse E358 centre (-216.7634, 46.7952) end of major axis (-217.6134, 46.7953) minor radius 0.8452 projected
  ellipse E359 centre (-211.6834, 46.7949) end of major axis (-213.6834, 46.795) minor radius 1.9887 projected
  ellipse E360 centre (-206.6034, 46.7947) end of major axis (-207.4534, 46.7947) minor radius 0.8452 projected
  ellipse E361 centre (-196.4933, 49.3198) end of major axis (-197.2433, 49.3198) minor radius 0.7458 projected
  ellipse E362 centre (-197.7634, 46.7942) end of major axis (-198.6134, 46.7942) minor radius 0.8452 projected
  ellipse E363 centre (-168.6034, 46.7926) end of major axis (-169.4534, 46.7927) minor radius 0.8452 projected
  ellipse E364 centre (-173.6834, 46.7929) end of major axis (-175.6834, 46.793) minor radius 1.9887 projected
  ellipse E365 centre (-178.7634, 46.7932) end of major axis (-179.6134, 46.7932) minor radius 0.8452 projected
  ellipse E366 centre (-192.6834, 46.7939) end of major axis (-194.6834, 46.794) minor radius 1.9887 projected
  ellipse E367 centre (-158.4933, 49.3177) end of major axis (-159.2433, 49.3178) minor radius 0.7458 projected
  ellipse E368 centre (-216.4071, 72.6481) end of major axis (-217.9321, 72.6482) minor radius 1.5164 projected
  ellipse E369 centre (-202.5124, 65.687) end of major axis (-203.3624, 65.687) minor radius 0.8452 projected
  ellipse E370 centre (-194.8922, 70.7378) end of major axis (-195.6422, 70.7379) minor radius 0.7458 projected
  ellipse E371 centre (-197.4324, 65.6867) end of major axis (-199.4324, 65.6868) minor radius 1.9887 projected
  ellipse E372 centre (-159.4324, 65.6847) end of major axis (-161.4324, 65.6848) minor radius 1.9887 projected
  ellipse E373 centre (-164.5124, 65.685) end of major axis (-165.3624, 65.685) minor radius 0.8452 projected
  ellipse E374 centre (-156.8922, 70.7358) end of major axis (-157.6422, 70.7359) minor radius 0.7458 projected
  ellipse E375 centre (-175.8922, 70.7368) end of major axis (-176.6422, 70.7369) minor radius 0.7458 projected
  ellipse E376 centre (-173.3524, 65.6854) end of major axis (-174.2024, 65.6855) minor radius 0.8452 projected
  ellipse E377 centre (-216.4079, 57.4943) end of major axis (-218.4079, 57.4944) minor radius 1.9887 projected
  ellipse E378 centre (-190.1432, 51.8451) end of major axis (-190.8932, 51.8451) minor radius 0.7458 projected
  ellipse E379 centre (-202.1845, 27.9019) end of major axis (-204.1845, 27.902) minor radius 1.9887 projected
  ellipse E380 centre (-207.2645, 27.9022) end of major axis (-208.1145, 27.9022) minor radius 0.8452 projected
  ellipse E381 centre (-205.9943, 30.4277) end of major axis (-206.7443, 30.4278) minor radius 0.7458 projected
  ellipse E382 centre (-188.2645, 27.9012) end of major axis (-189.1145, 27.9012) minor radius 0.8452 projected
  ellipse E383 centre (-186.9943, 30.4267) end of major axis (-187.7443, 30.4268) minor radius 0.7458 projected
  ellipse E384 centre (-197.1045, 27.9016) end of major axis (-197.9545, 27.9017) minor radius 0.8452 projected
  ellipse E385 centre (-164.1845, 27.8999) end of major axis (-166.1845, 27.9) minor radius 1.9887 projected
  ellipse E386 centre (-167.9943, 30.4257) end of major axis (-168.7443, 30.4257) minor radius 0.7458 projected
  ellipse E387 centre (-183.1845, 27.9009) end of major axis (-185.1845, 27.901) minor radius 1.9887 projected
  ellipse E388 centre (-178.1045, 27.9006) end of major axis (-178.9545, 27.9007) minor radius 0.8452 projected
  ellipse E389 centre (-211.6569, 76.3866) end of major axis (-213.6569, 76.3867) minor radius 1.9887 projected
  ellipse E390 centre (-167.5044, -6.5857) end of major axis (-167.7544, -6.5857) minor radius 0.2486 projected
  ellipse E391 centre (-168.9362, -5.1618) end of major axis (-170.2862, -5.1617) minor radius 1.3424 projected
  ellipse E392 centre (-170.3682, -6.5855) end of major axis (-170.6182, -6.5855) minor radius 0.2486 projected
  ellipse E393 centre (-167.5043, -3.7381) end of major axis (-167.7543, -3.7381) minor radius 0.2486 projected
  ellipse E394 centre (-166.9112, -5.1619) end of major axis (-167.1612, -5.1619) minor radius 0.2486 projected
  ellipse E395 centre (-159.766, -0.4392) end of major axis (-160.616, -0.4391) minor radius 0.8452 projected
  ellipse E396 centre (-170.9612, -5.1617) end of major axis (-171.2112, -5.1617) minor radius 0.2486 projected
  ellipse E397 centre (-197.106, -0.4372) end of major axis (-197.956, -0.4371) minor radius 0.8452 projected
  ellipse E398 centre (-188.266, -0.4376) end of major axis (-189.116, -0.4376) minor radius 0.8452 projected
  ellipse E399 centre (-216.106, -0.4362) end of major axis (-216.956, -0.4361) minor radius 0.8452 projected
  ellipse E400 centre (-207.266, -0.4366) end of major axis (-208.116, -0.4366) minor radius 0.8452 projected
  ellipse E401 centre (-202.186, -0.4369) end of major axis (-204.186, -0.4368) minor radius 1.9887 projected
  ellipse E402 centre (-158.4958, 2.0864) end of major axis (-159.2458, 2.0864) minor radius 0.7458 projected
  ellipse E403 centre (-186.9958, 2.0879) end of major axis (-187.7458, 2.088) minor radius 0.7458 projected
  ellipse E404 centre (-183.186, -0.4379) end of major axis (-185.186, -0.4378) minor radius 1.9887 projected
  ellipse E405 centre (-178.106, -0.4382) end of major axis (-178.956, -0.4381) minor radius 0.8452 projected
  ellipse E406 centre (-218.6457, 4.6152) end of major axis (-219.3957, 4.6153) minor radius 0.7458 projected
  ellipse E407 centre (-199.6457, 4.6142) end of major axis (-200.3957, 4.6143) minor radius 0.7458 projected
  ellipse E408 centre (-218.7849, 19.7094) end of major axis (-220.7849, 19.7095) minor radius 1.9887 projected
  ellipse E409 centre (-202.1809, 93.6777) end of major axis (-202.4309, 93.6778) minor radius 0.2486 projected
  ellipse E410 centre (-203.6129, 93.0881) end of major axis (-203.8629, 93.0881) minor radius 0.2486 projected
  ellipse E411 centre (-202.1812, 89.6507) end of major axis (-202.4312, 89.6507) minor radius 0.2486 projected
  ellipse E412 centre (-203.613, 90.2405) end of major axis (-203.863, 90.2405) minor radius 0.2486 projected
  ellipse E413 centre (-211.6561, 91.5404) end of major axis (-213.1811, 91.5405) minor radius 1.5164 projected
  ellipse E414 centre (-218.4764, 84.5804) end of major axis (-219.3264, 84.5804) minor radius 0.8452 projected
  ellipse E415 centre (-182.8514, 84.5785) end of major axis (-183.7014, 84.5785) minor radius 0.8452 projected
  ellipse E416 centre (-185.3912, 89.6299) end of major axis (-186.1412, 89.6299) minor radius 0.7458 projected
  ellipse E417 centre (-200.1561, 91.6641) end of major axis (-200.4061, 91.6641) minor radius 0.2486 projected
  ellipse E418 centre (-193.0114, 84.579) end of major axis (-193.8614, 84.5791) minor radius 0.8452 projected
  ellipse E419 centre (-200.7491, 93.0879) end of major axis (-200.9991, 93.0879) minor radius 0.2486 projected
  ellipse E420 centre (-200.7492, 90.2403) end of major axis (-200.9992, 90.2403) minor radius 0.2486 projected
  ellipse E421 centre (-168.9314, 84.5777) end of major axis (-170.9314, 84.5778) minor radius 1.9887 projected
  ellipse E422 centre (-208.9754, 103.4724) end of major axis (-209.8254, 103.4724) minor radius 0.8452 projected
  ellipse E423 centre (-195.3854, 103.4717) end of major axis (-196.2354, 103.4717) minor radius 0.8452 projected
  ellipse E424 centre (-194.1153, 105.9972) end of major axis (-194.8653, 105.9973) minor radius 0.7458 projected
  ellipse E425 centre (-219.1354, 103.4729) end of major axis (-219.9854, 103.473) minor radius 0.8452 projected
  ellipse E426 centre (-214.0554, 103.4727) end of major axis (-216.0554, 103.4728) minor radius 1.9887 projected
  ellipse E427 centre (-185.2254, 103.4711) end of major axis (-186.0754, 103.4712) minor radius 0.8452 projected
  ellipse E428 centre (-217.8653, 105.9985) end of major axis (-218.6153, 105.9985) minor radius 0.7458 projected
  ellipse E429 centre (-168.9363, -7.1754) end of major axis (-169.1863, -7.1753) minor radius 0.2486 projected
  ellipse E430 centre (97.8227, 106.1656) end of major axis (97.5727, 106.1656) minor radius 0.2486 projected
  ellipse E431 centre (23.4446, 103.46) end of major axis (21.4446, 103.4601) minor radius 1.9887 projected
  ellipse E432 centre (11.5697, 106.1702) end of major axis (11.3197, 106.1702) minor radius 0.2486 projected
  ellipse E433 centre (-4.1153, 105.9871) end of major axis (-4.8653, 105.9871) minor radius 0.7458 projected
  ellipse E434 centre (4.7746, 103.461) end of major axis (3.9246, 103.461) minor radius 0.8452 projected
  ellipse E435 centre (-18.9754, 103.4623) end of major axis (-19.8254, 103.4623) minor radius 0.8452 projected
  ellipse E436 centre (-154.6803, 106.1791) end of major axis (-154.9303, 106.1791) minor radius 0.2486 projected
  ellipse E437 centre (-153.2484, 106.7688) end of major axis (-153.4984, 106.7688) minor radius 0.2486 projected
  ellipse E438 centre (-110.9903, 105.9928) end of major axis (-111.7403, 105.9928) minor radius 0.7458 projected
  ellipse E439 centre (181.6268, 109.5985) end of major axis (181.3768, 109.5985) minor radius 0.2486 projected
  ellipse E440 centre (180.1947, 106.1612) end of major axis (179.9447, 106.1612) minor radius 0.2486 projected
  ellipse E441 centre (181.6266, 106.7509) end of major axis (181.3766, 106.7509) minor radius 0.2486 projected
  ellipse E442 centre (178.7629, 106.751) end of major axis (178.5129, 106.7511) minor radius 0.2486 projected
  ellipse E443 centre (180.1948, 108.1748) end of major axis (178.8448, 108.1748) minor radius 1.3424 projected
  ellipse E444 centre (178.763, 109.5986) end of major axis (178.513, 109.5986) minor radius 0.2486 projected
  ellipse E445 centre (178.1698, 108.1749) end of major axis (177.9198, 108.1749) minor radius 0.2486 projected
  ellipse E446 centre (173.3996, 103.452) end of major axis (172.5496, 103.452) minor radius 0.8452 projected
  ellipse E447 centre (164.5097, 105.9781) end of major axis (163.7597, 105.9781) minor radius 0.7458 projected
  ellipse E448 centre (163.2396, 103.4525) end of major axis (162.3896, 103.4526) minor radius 0.8452 projected
  ellipse E449 centre (168.3196, 103.4523) end of major axis (166.3196, 103.4524) minor radius 1.9887 projected
  ellipse E450 centre (170.8598, 108.5034) end of major axis (170.1098, 108.5034) minor radius 0.7458 projected
  ellipse E451 centre (145.5097, 105.9791) end of major axis (144.7597, 105.9791) minor radius 0.7458 projected
  ellipse E452 centre (149.3196, 103.4533) end of major axis (147.3196, 103.4534) minor radius 1.9887 projected
  ellipse E453 centre (151.8598, 108.5044) end of major axis (151.1098, 108.5044) minor radius 0.7458 projected
  ellipse E454 centre (154.3996, 103.453) end of major axis (153.5496, 103.453) minor radius 0.8452 projected
  ellipse E455 centre (96.3909, 106.7554) end of major axis (96.1409, 106.7554) minor radius 0.2486 projected
  ellipse E456 centre (97.8228, 108.1792) end of major axis (96.4728, 108.1792) minor radius 1.3424 projected
  ellipse E457 centre (96.391, 109.603) end of major axis (96.141, 109.603) minor radius 0.2486 projected
  ellipse E458 centre (99.2548, 109.6029) end of major axis (99.0048, 109.6029) minor radius 0.2486 projected
  ellipse E459 centre (99.2546, 106.7553) end of major axis (99.0046, 106.7553) minor radius 0.2486 projected
  ellipse E460 centre (99.8478, 108.179) end of major axis (99.5978, 108.1791) minor radius 0.2486 projected
  ellipse E461 centre (132.8598, 108.5054) end of major axis (132.1098, 108.5055) minor radius 0.7458 projected
  ellipse E462 centre (118.3197, 105.8413) end of major axis (116.7947, 105.8414) minor radius 1.5164 projected
  ellipse E463 centre (125.2396, 103.4546) end of major axis (124.3896, 103.4546) minor radius 0.8452 projected
  ellipse E464 centre (11.5698, 108.1838) end of major axis (10.2198, 108.1838) minor radius 1.3424 projected
  ellipse E465 centre (13.0018, 109.6075) end of major axis (12.7518, 109.6075) minor radius 0.2486 projected
  ellipse E466 centre (10.138, 109.6076) end of major axis (9.888, 109.6076) minor radius 0.2486 projected
  ellipse E467 centre (13.0016, 106.7599) end of major axis (12.7516, 106.7599) minor radius 0.2486 projected
  ellipse E468 centre (10.1379, 106.76) end of major axis (9.8879, 106.7601) minor radius 0.2486 projected
  ellipse E469 centre (13.5948, 108.1836) end of major axis (13.3448, 108.1837) minor radius 0.2486 projected
  ellipse E470 centre (19.6347, 105.9858) end of major axis (18.8847, 105.9859) minor radius 0.7458 projected
  ellipse E471 centre (25.9848, 108.5111) end of major axis (25.2348, 108.5112) minor radius 0.7458 projected
  ellipse E472 centre (64.7597, 105.9834) end of major axis (64.0097, 105.9835) minor radius 0.7458 projected
  ellipse E473 centre (52.1098, 108.5097) end of major axis (51.3598, 108.5098) minor radius 0.7458 projected
  ellipse E474 centre (45.7597, 105.9844) end of major axis (45.0097, 105.9845) minor radius 0.7458 projected
  ellipse E475 centre (54.6496, 103.4583) end of major axis (53.7996, 103.4584) minor radius 0.8452 projected
  ellipse E476 centre (63.4896, 103.4579) end of major axis (62.6396, 103.4579) minor radius 0.8452 projected
  ellipse E477 centre (44.4896, 103.4589) end of major axis (43.6396, 103.4589) minor radius 0.8452 projected
  ellipse E478 centre (92.6496, 103.4563) end of major axis (91.7996, 103.4563) minor radius 0.8452 projected
  ellipse E479 centre (87.5696, 103.4566) end of major axis (85.5696, 103.4567) minor radius 1.9887 projected
  ellipse E480 centre (83.7597, 105.9824) end of major axis (83.0097, 105.9824) minor radius 0.7458 projected
  ellipse E481 centre (73.6496, 103.4573) end of major axis (72.7996, 103.4574) minor radius 0.8452 projected
  ellipse E482 centre (82.4896, 103.4568) end of major axis (81.6396, 103.4569) minor radius 0.8452 projected
  ellipse E483 centre (90.1098, 108.5077) end of major axis (89.3598, 108.5077) minor radius 0.7458 projected
  ellipse E484 centre (68.5696, 103.4576) end of major axis (66.5696, 103.4577) minor radius 1.9887 projected